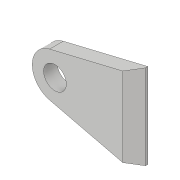
# Autodesk Inventor part: FRC003-1
Saved by Autodesk Inventor 2020 (Build 240168000, 168)
## iProperties
Created: 2020-02-07
Part Number: FRC003-1
Material: Generic
Document SubType Name: Modeling
Designer: Juan Carlos Botero
Density: 1 g/cm^3
Appearance: Default
Mass: 6.52409 g
Surface Area: 32.0611 cm^2
Volume: 6.52409 cm^3
Author: Juan Carlos Botero
Title: SOPORTE PIVOTE
Autodesk Inventor part; units mm, degrees
ref_plane "YZ Plane" through (0, 0, 0) normal (1, 0, 0) x (0, 1, 0)
ref_plane "XZ Plane" through (0, 0, 0) normal (0, 1, 0) x (-1, 0, 0)
ref_plane "XY Plane" through (0, 0, 0) normal (0, 0, 1) x (1, 0, 0)
sketch "Sketch1" plane through (0, 0, 0) normal (0, 0, 1) x (1, 0, 0)
  circle A0 centre (-790.1228, -10.9134) radius 9.525 projected
  ellipse E0 centre (61.5218, 18.65) end of major axis (52.5416, 18.65) minor radius 6.35 (61.5218, 25) -> (52.5416, 18.65) ccw
  line L0 (61.5218, 25) -> (114.272, 25)
  ellipse E1 centre (114.272, 18.65) end of major axis (105.2917, 18.65) minor radius 6.35 (123.2522, 18.65) -> (114.272, 25) ccw
  line L1 (123.2522, 18.65) -> (123.2522, -18.65)
  ellipse E2 centre (114.272, -18.65) end of major axis (105.2917, -18.65) minor radius 6.35 (114.272, -25) -> (123.2522, -18.65) ccw
  line L2 (114.272, -25) -> (61.5218, -25)
  ellipse E3 centre (61.5218, -18.65) end of major axis (52.5416, -18.65) minor radius 6.35 (52.5416, -18.65) -> (61.5218, -25) ccw
  line L3 (52.5416, -18.65) -> (52.5416, 18.65)
  line L4 (114.272, 21.825) -> (61.5218, 21.825)
  ellipse E4 centre (61.5218, 18.65) end of major axis (57.0317, 18.65) minor radius 3.175 (61.5218, 21.825) -> (57.0317, 18.65) ccw
  line L5 (57.0317, 18.65) -> (57.0317, -18.65)
  ellipse E5 centre (61.5218, -18.65) end of major axis (57.0317, -18.65) minor radius 3.175 (57.0317, -18.65) -> (61.5218, -21.825) ccw
  line L6 (61.5218, -21.825) -> (114.272, -21.825)
  ellipse E6 centre (114.272, -18.65) end of major axis (109.7818, -18.65) minor radius 3.175 (114.272, -21.825) -> (118.7621, -18.65) ccw
  line L7 (118.7621, -18.65) -> (118.7621, 18.65)
  ellipse E7 centre (114.272, 18.65) end of major axis (109.7818, 18.65) minor radius 3.175 (118.7621, 18.65) -> (114.272, 21.825) ccw
  circle A1 centre (17.6912, 0) radius 5 projected
  circle A2 centre (17.6912, 0) radius 10
  line L8 (15.357, 9.7238) -> (52.5416, 18.65)
  line L9 (52.5416, -18.65) -> (15.357, -9.7238)
  dimension "d4" = 20
  constraints: 20 end point, 4 horizontal, 4 vertical, 2 point on circle, 2 tangent, 1 centre point, 1 coincident, 56 other
  measures "d4" diameter of A2
extrude "Extrusion1" add sketch "Sketch1" along normal blind 6 contours L3 L9 A2 L8 | A2
chamfer "Chamfer1" distance 5 angle 45 1 edges at (52.5416, 0, 6)
body "Solid1"
